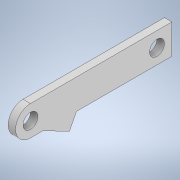
# Autodesk Inventor part: IntakeBraket
Saved by Autodesk Inventor 2021 (Build 250183000, 183)
## iProperties
Created: 2021-01-12
Part Number: IntakeBraket
Material: Generic
Document SubType Name: Modeling
Designer: User
Density: 1 g/cm^3
Appearance: Default
Author: User
Autodesk Inventor part; units mm, degrees
ref_plane "YZ Plane" through (0, 0, 0) normal (1, 0, 0) x (0, 1, 0)
ref_plane "XZ Plane" through (0, 0, 0) normal (0, 1, 0) x (-1, 0, 0)
ref_plane "XY Plane" through (0, 0, 0) normal (0, 0, 1) x (1, 0, 0)
sketch "Sketch1" plane through (0, 0, 0) normal (1, 0, 0) x (0, 1, 0)
  line L0 (0, 0) -> (25.4, 0)
  line L1 (25.4, 0) -> (25.4, -133.35)
  line L2 (25.4, -133.35) -> (0, -133.35)
  line L3 (0, -133.35) -> (0, 0)
  dimension "d0" = 25.4
  dimension "d1" = 133.35
  constraints: 8 end point, 2 parallel, 1 horizontal, 1 perpendicular
  measures "d0" distance of L1.end L2.end
  measures "d1" distance of L0.end L1.end
extrude "Extrusion1" add sketch "Sketch1" along normal blind 6.35
sketch "Sketch2" plane through (6.35, 0, 0) normal (1, 0, 0) x (0, 0, -1)
  line L0 (133.35, 0) -> (133.35, 25.4) projected
  line L1 (133.35, 25.4) -> (0, 25.4) projected
  line L2 (0, 25.4) -> (0, 0) projected
  line L3 (0, 0) -> (133.35, 0) projected
  circle A0 centre (12.7, 12.7) radius 6.35
  circle A1 centre (120.65, 12.7) radius 6.35
  dimension "d4" = 25.4
  dimension "d5" = 12.7
  dimension "d6" = 12.7
  dimension "d7" = 107.95
  dimension "d8" = 133.35
  dimension "d9" = 12.7
  dimension "d10" = 12.7
  dimension "d11" = 12.7
  constraints: 2 centre point, 2 coincident
  measures "d4" distance of L0.start L0.end
  measures "d5" distance from line of L1 point (120.65, 12.7)
  measures "d6" distance from line of L1 point (12.7, 12.7)
  measures "d7" distance of point (120.65, 12.7) point (12.7, 12.7)
  measures "d8" distance between parallel lines of L0 L2
  measures "d9" distance from line of point (12.7, 12.7) L2
  measures "d10" diameter of A0
  measures "d11" diameter of A1
extrude "Extrusion2" cut sketch "Sketch2" against normal blind 6.35 contours A0 | A1
sketch "Sketch3" plane through (6.35, 0, 0) normal (1, 0, 0) x (0, 0, -1)
  circle A0 centre (12.7, 12.7) radius 6.35 projected
  circle A1 centre (12.7, 12.7) radius 12.7
  line L0 (133.35, 25.4) -> (0, 25.4) projected
  line L1 (0, 25.4) -> (0, 0) projected
  line L2 (0, 0) -> (133.35, 0) projected
  point P0 (12.7, 0)
  point P1 (0, 12.7)
  point P2 (12.7, 25.4)
  constraints: 3 tangent, 1 centre point, 1 coincident
extrude "Extrusion3" cut sketch "Sketch3" against normal blind 6.35 contours A1 L1 L0 | L2 L1 A1
sketch "Sketch4" plane through (6.35, 0, 0) normal (1, 0, 0) x (0, 0, -1)
  circle A0 centre (12.7, 12.7) radius 6.35 projected
  line L0 (120.65, 12.7) -> (12.7, 12.7)
  circle A1 centre (120.65, 12.7) radius 6.35 projected
  line L1 (12.7, 12.7) -> (120.65, -43.3755)
  line L2 (120.65, -43.3755) -> (120.65, 12.7)
  line L3 (12.7, 12.7) -> (9.7728, 7.0649)
  line L4 (9.7728, 7.0649) -> (45.9137, -11.7087)
  line L5 (45.9137, -11.7087) -> (48.8409, -6.0737)
  line L6 (12.7, 0) -> (133.35, 0) projected
  line L7 (48.8409, -6.0737) -> (51.9959, 0)
  point P0 (0, 0)
  point P1 (23.3734, 0)
  dimension "d16" = 27.45
  dimension "d19" = 25.4
  constraints: 14 end point, 4 point on line, 3 perpendicular, 2 coincident, 1 horizontal, 1 parallel, 1 vertical, 2 other
  measures "d16" angle of L0 L1
  measures "d19" distance from line of L5 point (23.373, 0)
extrude "Extrusion4" add sketch "Sketch4" against normal blind 6.35 contours L6 L1 L5 L4 | L6 L7 L1
equation "\"d5\" = 0.5 * d4"
equation "\"d6\" = d5"
equation "\"d9\" = -0.5 * d7 + 0.5 * d8"
body "Solid1"
